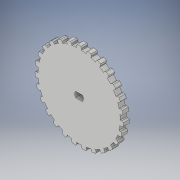
# Autodesk Inventor part: Hybrid Driver Gear
Saved by Autodesk Inventor 2017 (Build 210142000, 142)
## iProperties
Created: 2018-03-08
Part Number: Hybrid Driver Gear
Material: Generic
Document SubType Name: Modeling
Designer: Russ
Density: 1 g/cm^3
Appearance: Default
Author: Russ
Autodesk Inventor part; units mm, degrees
ref_plane "YZ Plane" through (0, 0, 0) normal (1, 0, 0) x (0, 1, 0)
ref_plane "XZ Plane" through (0, 0, 0) normal (0, 1, 0) x (-1, 0, 0)
ref_plane "XY Plane" through (0, 0, 0) normal (0, 0, 1) x (1, 0, 0)
sketch "Sketch1" plane through (0, 0, 0) normal (0, 0, 1) x (1, 0, 0)
  arc A0 (-1.4953, 25.674) -> (1.4953, 25.674) centre (0, 0) ccw
  line L0 (0, 25.7175) -> (0, 27.6225)
  line L1 (0, 27.6225) -> (1.016, 27.6225)
  line L2 (0, 27.6225) -> (-1.016, 27.6225)
  line L3 (-1.4953, 25.674) -> (-1.6061, 27.5758)
  line L4 (-2.9856, 25.5436) -> (-3.2068, 27.4357)
  line L5 (-4.4658, 25.3268) -> (-4.7966, 27.2029)
  line L6 (-5.9309, 25.0243) -> (-6.3702, 26.8779)
  line L7 (-7.3759, 24.6371) -> (-7.9222, 26.4621)
  line L8 (-8.7959, 24.1665) -> (-9.4475, 25.9567)
  line L9 (-10.1862, 23.6142) -> (-10.9407, 25.3634)
  line L10 (-11.542, 22.982) -> (-12.397, 24.6844)
  line L11 (-12.8587, 22.272) -> (-13.8112, 23.9218)
  line L12 (-14.132, 21.4867) -> (-15.1788, 23.0783)
  line L13 (-15.3574, 20.6286) -> (-16.495, 22.1566)
  line L14 (-16.5309, 19.7007) -> (-17.7554, 21.1601)
  line L15 (-17.6484, 18.7062) -> (-18.9557, 20.0919)
  line L16 (-18.7062, 17.6484) -> (-20.0919, 18.9557)
  line L17 (-19.7007, 16.5309) -> (-21.1601, 17.7554)
  line L18 (-20.6286, 15.3574) -> (-22.1566, 16.495)
  line L19 (-21.4867, 14.132) -> (-23.0783, 15.1788)
  line L20 (-22.272, 12.8588) -> (-23.9218, 13.8113)
  line L21 (-22.982, 11.542) -> (-24.6844, 12.397)
  line L22 (-23.6142, 10.1862) -> (-25.3634, 10.9407)
  line L23 (-24.1665, 8.7959) -> (-25.9567, 9.4475)
  line L24 (-24.6371, 7.3759) -> (-26.4621, 7.9222)
  line L25 (-25.0243, 5.9309) -> (-26.8779, 6.3702)
  line L26 (-25.3268, 4.4658) -> (-27.2029, 4.7966)
  line L27 (-25.5436, 2.9856) -> (-27.4357, 3.2068)
  line L28 (-25.674, 1.4953) -> (-27.5758, 1.6061)
  line L29 (-25.7175, 0) -> (-27.6225, 0)
  line L30 (-25.674, -1.4953) -> (-27.5758, -1.6061)
  line L31 (-25.5436, -2.9856) -> (-27.4357, -3.2068)
  line L32 (-25.3268, -4.4658) -> (-27.2029, -4.7966)
  line L33 (-25.0243, -5.9309) -> (-26.8779, -6.3702)
  line L34 (-24.6371, -7.3759) -> (-26.4621, -7.9222)
  line L35 (-24.1665, -8.7959) -> (-25.9567, -9.4475)
  line L36 (-23.6142, -10.1862) -> (-25.3634, -10.9407)
  line L37 (-22.982, -11.542) -> (-24.6844, -12.397)
  line L38 (-22.272, -12.8587) -> (-23.9218, -13.8112)
  line L39 (-21.4867, -14.132) -> (-23.0783, -15.1788)
  line L40 (-20.6286, -15.3574) -> (-22.1566, -16.495)
  line L41 (-19.7007, -16.5309) -> (-21.1601, -17.7554)
  line L42 (-18.7062, -17.6484) -> (-20.0919, -18.9557)
  line L43 (-17.6484, -18.7062) -> (-18.9557, -20.0919)
  line L44 (-16.5309, -19.7007) -> (-17.7554, -21.1601)
  line L45 (-15.3574, -20.6286) -> (-16.495, -22.1566)
  line L46 (-14.132, -21.4867) -> (-15.1788, -23.0783)
  line L47 (-12.8587, -22.272) -> (-13.8112, -23.9218)
  line L48 (-11.542, -22.982) -> (-12.397, -24.6844)
  line L49 (-10.1862, -23.6142) -> (-10.9407, -25.3634)
  line L50 (-8.7959, -24.1665) -> (-9.4475, -25.9567)
  line L51 (-7.3759, -24.6371) -> (-7.9222, -26.4621)
  line L52 (-5.9309, -25.0243) -> (-6.3702, -26.8779)
  line L53 (-4.4658, -25.3268) -> (-4.7966, -27.2029)
  line L54 (-2.9856, -25.5436) -> (-3.2068, -27.4357)
  line L55 (-1.4953, -25.674) -> (-1.6061, -27.5758)
  line L56 (0, -25.7175) -> (0, -27.6225)
  line L57 (1.4953, -25.674) -> (1.6061, -27.5758)
  line L58 (2.9856, -25.5436) -> (3.2068, -27.4357)
  line L59 (4.4658, -25.3268) -> (4.7966, -27.2029)
  line L60 (5.9309, -25.0243) -> (6.3702, -26.8779)
  line L61 (7.3759, -24.6371) -> (7.9222, -26.4621)
  line L62 (8.7959, -24.1665) -> (9.4475, -25.9567)
  line L63 (10.1862, -23.6142) -> (10.9407, -25.3634)
  line L64 (11.542, -22.982) -> (12.397, -24.6844)
  line L65 (12.8588, -22.272) -> (13.8113, -23.9218)
  line L66 (14.132, -21.4867) -> (15.1788, -23.0783)
  line L67 (15.3574, -20.6286) -> (16.495, -22.1566)
  line L68 (16.5309, -19.7007) -> (17.7554, -21.1601)
  line L69 (17.6484, -18.7062) -> (18.9557, -20.0919)
  line L70 (18.7062, -17.6484) -> (20.0919, -18.9557)
  line L71 (19.7007, -16.5309) -> (21.1601, -17.7554)
  line L72 (20.6286, -15.3574) -> (22.1566, -16.495)
  line L73 (21.4867, -14.132) -> (23.0783, -15.1788)
  line L74 (22.272, -12.8588) -> (23.9218, -13.8113)
  line L75 (22.982, -11.542) -> (24.6844, -12.397)
  line L76 (23.6142, -10.1862) -> (25.3634, -10.9407)
  line L77 (24.1665, -8.7959) -> (25.9567, -9.4475)
  line L78 (24.6371, -7.3759) -> (26.4621, -7.9222)
  line L79 (25.0243, -5.9309) -> (26.8779, -6.3702)
  line L80 (25.3268, -4.4658) -> (27.2029, -4.7966)
  line L81 (25.5436, -2.9856) -> (27.4357, -3.2068)
  line L82 (25.674, -1.4953) -> (27.5758, -1.6061)
  line L83 (25.7175, 0) -> (27.6225, 0)
  line L84 (25.674, 1.4953) -> (27.5758, 1.6061)
  line L85 (25.5436, 2.9856) -> (27.4357, 3.2068)
  line L86 (25.3268, 4.4658) -> (27.2029, 4.7966)
  line L87 (25.0243, 5.9309) -> (26.8779, 6.3702)
  line L88 (24.6371, 7.3759) -> (26.4621, 7.9222)
  line L89 (24.1665, 8.7959) -> (25.9567, 9.4475)
  line L90 (23.6142, 10.1862) -> (25.3634, 10.9407)
  line L91 (22.982, 11.542) -> (24.6844, 12.397)
  line L92 (22.272, 12.8588) -> (23.9218, 13.8113)
  line L93 (21.4867, 14.132) -> (23.0783, 15.1788)
  line L94 (20.6286, 15.3574) -> (22.1566, 16.495)
  line L95 (19.7007, 16.5309) -> (21.1601, 17.7554)
  line L96 (18.7062, 17.6484) -> (20.0919, 18.9557)
  line L97 (17.6484, 18.7062) -> (18.9557, 20.0919)
  line L98 (16.5309, 19.7007) -> (17.7554, 21.1601)
  line L99 (15.3574, 20.6286) -> (16.495, 22.1566)
  line L100 (14.132, 21.4867) -> (15.1788, 23.0783)
  line L101 (12.8588, 22.272) -> (13.8113, 23.9218)
  line L102 (11.542, 22.982) -> (12.397, 24.6844)
  line L103 (10.1862, 23.6142) -> (10.9407, 25.3634)
  line L104 (8.7959, 24.1665) -> (9.4475, 25.9567)
  line L105 (7.3759, 24.6371) -> (7.9222, 26.4621)
  line L106 (5.9309, 25.0243) -> (6.3702, 26.8779)
  line L107 (4.4658, 25.3268) -> (4.7966, 27.2029)
  line L108 (2.9856, 25.5436) -> (3.2068, 27.4357)
  line L109 (1.4953, 25.674) -> (1.6061, 27.5758)
  arc A1 (-1.016, 27.6225) -> (-1.5507, 26.6249) centre (0.0119, 26.4294) ccw
  arc A2 (1.5507, 26.6249) -> (1.016, 27.6225) centre (-0.0119, 26.4294) ccw
  dimension "d0" = 51.435
  dimension "d4" = 1.905
  dimension "d5" = 1.016
  dimension "d6" = 1.016
  dimension "d9" = 360
  dimension "d11" = 1.5748
  dimension "d12" = 1.5748
  constraints: 220 end point, 6 point on circle, 3 centre point, 2 horizontal, 2 midpoint, 1 coincident, 1 vertical, 325 other
  measures "d0" diameter of A0
  measures "d4" distance of L0.start L0.end
  measures "d5" distance of L0.end L1.end
  measures "d6" distance of L0.end L2.end
  measures "d11" radius of A1
  measures "d12" radius of A2
extrude "Extrusion1" add sketch "Sketch1" along normal blind 3.81
pattern_circular "Circular Pattern1" count 27 over 360 about axis through (0, 0, 0) along (0, 0, 1) of "Extrusion1"
sketch "Sketch2" plane through (0, 0, 3.81) normal (0, 0, 1) x (1, 0, 0)
  line L0 (0, 0) -> (0, 1.6891)
  line L1 (0, 1.6891) -> (2.1454, 1.6891)
  line L2 (0, 1.6891) -> (-2.1454, 1.6891)
  line L3 (0, 0) -> (0.1755, 0)
  line L4 (0, -1.6891) -> (-2.1454, -1.6891)
  line L5 (0, -1.6891) -> (2.1454, -1.6891)
  arc A0 (-2.1454, 1.6891) -> (-2.1454, -1.6891) centre (0, 0) ccw
  arc A1 (2.1454, -1.6891) -> (2.1454, 1.6891) centre (0, 0) ccw
  circle A2 centre (0, 0) radius 2.7305
  dimension "d23" = 3.3782
  dimension "d24" = 5.461
  dimension "d25" = 0
  constraints: 12 end point, 4 point on circle, 4 symmetric about line, 3 centre point, 2 coincident, 1 concentric, 1 horizontal, 1 perpendicular, 1 vertical
  measures "d23" distance between parallel lines of L5 L1
  measures "d24" diameter of A2
  measures "d25" distance of point (0, 0) point (0, 0)
extrude "Extrusion2" cut sketch "Sketch2" against normal up to next contours L1 A1 L5 L4 A0 L2
sketch "Sketch4" plane through (0, 0, 0) normal (0, 0, -1) x (-1, 0, 0)
  arc A0 (-2, 1.5) -> (-2, -1.5) centre (0, 0) ccw
  line L0 (-2, 1.5) -> (2, 1.5)
  arc A1 (2, -1.5) -> (2, 1.5) centre (0, 0) ccw
  line L1 (2, -1.5) -> (-2, -1.5)
  line L2 (1.4866, 7.4736) -> (1.6724, 8.4079)
  arc A2 (1.6724, 8.4079) -> (1.016, 9.525) centre (0.1056, 8.2386) ccw
  line L3 (1.016, 9.525) -> (-1.016, 9.525)
  arc A3 (-1.016, 9.525) -> (-1.6724, 8.4079) centre (-0.1056, 8.2386) ccw
  line L4 (-1.6724, 8.4079) -> (-1.4866, 7.4736)
  arc A4 (-1.4866, 7.4736) -> (-4.2334, 6.3358) centre (0, 0) ccw
  line L5 (-4.2334, 6.3358) -> (-4.7627, 7.1279)
  arc A5 (-4.7627, 7.1279) -> (-6.0168, 7.4536) centre (-5.7509, 5.9002) ccw
  line L6 (-6.0168, 7.4536) -> (-7.4536, 6.0168)
  arc A6 (-7.4536, 6.0168) -> (-7.1279, 4.7627) centre (-5.9002, 5.7509) ccw
  line L7 (-7.1279, 4.7627) -> (-6.3358, 4.2334)
  arc A7 (-6.3358, 4.2334) -> (-7.4736, 1.4866) centre (0, 0) ccw
  line L8 (-7.4736, 1.4866) -> (-8.4079, 1.6724)
  arc A8 (-8.4079, 1.6724) -> (-9.525, 1.016) centre (-8.2386, 0.1056) ccw
  line L9 (-9.525, 1.016) -> (-9.525, -1.016)
  arc A9 (-9.525, -1.016) -> (-8.4079, -1.6724) centre (-8.2386, -0.1056) ccw
  line L10 (-8.4079, -1.6724) -> (-7.4736, -1.4866)
  arc A10 (-7.4736, -1.4866) -> (-6.3358, -4.2334) centre (0, 0) ccw
  line L11 (-6.3358, -4.2334) -> (-7.1279, -4.7627)
  arc A11 (-7.1279, -4.7627) -> (-7.4536, -6.0168) centre (-5.9002, -5.7509) ccw
  line L12 (-7.4536, -6.0168) -> (-6.0168, -7.4536)
  arc A12 (-6.0168, -7.4536) -> (-4.7627, -7.1279) centre (-5.7509, -5.9002) ccw
  line L13 (-4.7627, -7.1279) -> (-4.2334, -6.3358)
  arc A13 (-4.2334, -6.3358) -> (-1.4866, -7.4736) centre (0, 0) ccw
  line L14 (-1.4866, -7.4736) -> (-1.6724, -8.4079)
  arc A14 (-1.6724, -8.4079) -> (-1.016, -9.525) centre (-0.1056, -8.2386) ccw
  line L15 (-1.016, -9.525) -> (1.016, -9.525)
  arc A15 (1.016, -9.525) -> (1.6724, -8.4079) centre (0.1056, -8.2386) ccw
  line L16 (1.6724, -8.4079) -> (1.4866, -7.4736)
  arc A16 (1.4866, -7.4736) -> (4.2334, -6.3358) centre (0, 0) ccw
  line L17 (4.2334, -6.3358) -> (4.7627, -7.1279)
  arc A17 (4.7627, -7.1279) -> (6.0168, -7.4536) centre (5.7509, -5.9002) ccw
  line L18 (6.0168, -7.4536) -> (7.4536, -6.0168)
  arc A18 (7.4536, -6.0168) -> (7.1279, -4.7627) centre (5.9002, -5.7509) ccw
  line L19 (7.1279, -4.7627) -> (6.3358, -4.2334)
  arc A19 (6.3358, -4.2334) -> (7.4736, -1.4866) centre (0, 0) ccw
  line L20 (7.4736, -1.4866) -> (8.4079, -1.6724)
  arc A20 (8.4079, -1.6724) -> (9.525, -1.016) centre (8.2386, -0.1056) ccw
  line L21 (9.525, -1.016) -> (9.525, 1.016)
  arc A21 (9.525, 1.016) -> (8.4079, 1.6724) centre (8.2386, 0.1056) ccw
  line L22 (8.4079, 1.6724) -> (7.4736, 1.4866)
  arc A22 (7.4736, 1.4866) -> (6.3358, 4.2334) centre (0, 0) ccw
  line L23 (6.3358, 4.2334) -> (7.1279, 4.7627)
  arc A23 (7.1279, 4.7627) -> (7.4536, 6.0168) centre (5.9002, 5.7509) ccw
  line L24 (7.4536, 6.0168) -> (6.0168, 7.4536)
  arc A24 (6.0168, 7.4536) -> (4.7627, 7.1279) centre (5.7509, 5.9002) ccw
  line L25 (4.7627, 7.1279) -> (4.2334, 6.3358)
  arc A25 (4.2334, 6.3358) -> (1.4866, 7.4736) centre (0, 0) ccw
  constraints: 52 end point, 52 point on circle, 26 centre point
extrude "Extrusion3" add sketch "Sketch4" along normal blind 9.81
body "Solid1"
